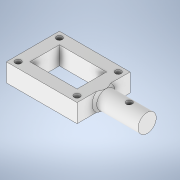
# Autodesk Inventor part: MotorHolder
Saved by Autodesk Inventor 2022.1 (Build 261234020, 234B)
## iProperties
Created: 2021-11-05
Part Number: MotorHolder
Material: ABS Plastic
Document SubType Name: Modeling
Designer: Alexander
Density: 1.06 g/cm^3
Appearance: Smooth - White
Mass: 21.2129 g
Surface Area: 88.1603 cm^2
Volume: 20.0122 cm^3
Author: Alexander
Autodesk Inventor part; units mm, degrees
ref_plane "YZ Plane" through (0, 0, 0) normal (1, 0, 0) x (0, 1, 0)
ref_plane "XZ Plane" through (0, 0, 0) normal (0, 1, 0) x (-1, 0, 0)
ref_plane "XY Plane" through (0, 0, 0) normal (0, 0, 1) x (1, 0, 0)
sketch "Sketch3" plane through (0, 0, 0) normal (0, 1, 0) x (-1, 0, 0)
  line L0 (-30, -22.5) -> (30, -22.5)
  line L1 (30, -22.5) -> (30, 22.5)
  line L2 (30, 22.5) -> (-30, 22.5)
  line L3 (-30, 22.5) -> (-30, -22.5)
  line L4 (-30, -22.5) -> (30, 22.5) construction
  line L5 (30, -22.5) -> (-30, 22.5) construction
  circle A0 centre (-25, 17.5) radius 2.5
  circle A1 centre (25, 17.5) radius 2.5
  circle A2 centre (-25, -17.5) radius 2.5
  circle A3 centre (25, -17.5) radius 2.5
  line L6 (-20, -12.5) -> (20, -12.5)
  line L7 (20, -12.5) -> (20, 12.5)
  line L8 (20, 12.5) -> (-20, 12.5)
  line L9 (-20, 12.5) -> (-20, -12.5)
  line L10 (-20, -12.5) -> (20, 12.5) construction
  line L11 (20, -12.5) -> (-20, 12.5) construction
  point P0 (0, 0)
  dimension "d31" = 60
  dimension "d32" = 45
  dimension "d39" = 5
  dimension "d40" = 5
  dimension "d41" = 5
  dimension "d44" = 50
  dimension "d47" = 35
  dimension "d50" = 40
  dimension "d51" = 25
  constraints: 24 end point, 4 centre point, 4 midpoint, 4 parallel, 3 horizontal, 2 perpendicular, 1 vertical, 6 other
  measures "d31" distance of L2.end L1.end
  measures "d32" distance of L1.end L0.end
  measures "d39" diameter of A0
  measures "d40" distance from line of L3 A0.centre
  measures "d41" distance from line of L2 A0.centre
  measures "d44" distance of A0.centre A1.centre
  measures "d47" distance of A0.centre A2.centre
  measures "d50" distance of L8.end L7.end
  measures "d51" distance of L7.end L6.end
extrude "Extrusion3" add sketch "Sketch3" along normal blind 15.5
sketch "Sketch4" plane through (-30, 0, -22.5) normal (-1, 0, 0) x (0, 0, 1)
  line L0 (0, 15.5) -> (45, 15.5) projected
  circle A0 centre (22.5, 7.75) radius 7.75
  line L1 (0, 0) -> (0, 15.5) projected
  line L2 (0, 0) -> (45, 0) projected
  point P0 (22.5, 0)
  dimension "d76" = 15.5
  dimension "d77" = 22.5
  dimension "d78" = 7.75
  dimension "d82" = 15.5
  constraints: 1 centre point
  measures "d76" diameter of A0
  measures "d77" distance from line of L1 A0.centre
  measures "d78" distance from line of L2 A0.centre
  measures "d82" distance between parallel lines of L0 L2
extrude "Extrusion4" add sketch "Sketch4" along normal blind 37 contours A0
sketch "Sketch7" plane through (0, 0, 0) normal (0, -1, 0) x (1, 0, 0)
  circle A0 centre (-52, 0) radius 2.5
  line L0 (-30, -22.5) -> (-30, 22.5) projected
  point P0 (0, 0)
  point P1 (-30, 0)
  dimension "d69" = 5
  dimension "d70" = 22
  constraints: 1 centre point
  measures "d69" diameter of A0
  measures "d70" distance from line of L0 A0.centre
extrude "Extrusion7" cut sketch "Sketch7" against normal through all
chamfer "Chamfer2" distance 2 angle 45 3 edges at (-30, 7.75, -7.75) (-30, 13.2301, 5.4801) (-30, 2.2699, 5.4801)
equation "\"d76\" = d82"
equation "\"d78\" = 0.5 * d76"
body "Solid2"
